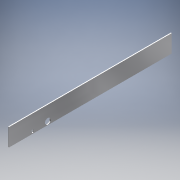
# Autodesk Inventor part: Bumper Plate
Saved by Autodesk Inventor 2019 (Build 230136000, 136)
## iProperties
Created: 2019-10-20
Part Number: Bumper Plate
Material: Aluminum 6061
Document SubType Name: Modeling
Designer: admin
Density: 2.7 g/cm^3
Appearance: Aluminum - Flat
Author: admin
Autodesk Inventor part; units mm, degrees
ref_plane "YZ Plane" through (0, 0, 0) normal (1, 0, 0) x (0, 1, 0)
ref_plane "XZ Plane" through (0, 0, 0) normal (0, 1, 0) x (-1, 0, 0)
ref_plane "XY Plane" through (0, 0, 0) normal (0, 0, 1) x (1, 0, 0)
sketch "Sketch1" plane through (0, 0, 0) normal (1, 0, 0) x (0, 1, 0)
  line L0 (-50, 460) -> (50, 460)
  line L1 (50, 460) -> (50, -460)
  line L2 (50, -460) -> (-50, -460)
  line L3 (-50, -460) -> (-50, 460)
  line L4 (-50, 460) -> (50, -460) construction
  line L5 (50, 460) -> (-50, -460) construction
  point P0 (0, 0)
  dimension "d0" = 920
  dimension "d1" = 100
  constraints: 12 end point, 2 midpoint, 2 parallel, 1 horizontal, 1 perpendicular
  measures "d0" distance of L0.end L1.end
  measures "d1" distance of L0.start L0.end
extrude "Extrusion1" add sketch "Sketch1" along normal blind 5
sketch "Sketch2" plane through (5, 0, 0) normal (1, 0, 0) x (0, 0, -1)
  circle A0 centre (-240.911, -31.452) radius 12.25
  line L0 (-460, -50) -> (460, -50) projected
  line L1 (-460, 50) -> (-460, -50) projected
  point P0 (0, 0)
  dimension "d4" = 24.5
  dimension "d5" = 18.548
  dimension "d8" = 219.089
  constraints: 1 centre point
  measures "d4" diameter of A0
  measures "d5" distance from line of L0 A0.centre
  measures "d8" distance from line of L1 A0.centre
extrude "Extrusion2" cut sketch "Sketch2" against normal through all
sketch "Sketch3" plane through (5, 0, 0) normal (1, 0, 0) x (0, 0, -1)
  arc A0 (-321.8744, -41.3708) -> (-330.8076, -42.4652) centre (-326.341, -41.918) ccw construction
  line L0 (-460, 50) -> (-460, -50) projected
  line L1 (-460, -50) -> (460, -50) projected
  circle A1 centre (-240.911, -31.452) radius 12.25 projected
  arc A2 (-326.9797, -31.4287) -> (-326.341, -41.918) centre (-240.911, -31.452) ccw construction
  arc A3 (-326.8633, -35.9272) -> (-322.4797, -31.4299) centre (-326.9797, -31.4287) ccw construction
  line L2 (-326.9797, -31.4287) -> (-240.911, -31.452) construction
  line L3 (-240.911, -31.452) -> (-326.341, -41.918) construction
  arc A4 (-331.4797, -31.4275) -> (-330.8076, -42.4652) centre (-240.911, -31.452) ccw
  arc A5 (-322.4797, -31.4299) -> (-321.8744, -41.3708) centre (-240.911, -31.452) ccw
  arc A6 (-330.8076, -42.4652) -> (-321.8744, -41.3708) centre (-326.341, -41.918) ccw
  arc A7 (-331.4797, -31.4275) -> (-326.8633, -35.9272) centre (-326.9797, -31.4287) ccw construction
  arc A8 (-322.4797, -31.4299) -> (-331.4797, -31.4275) centre (-326.9797, -31.4287) ccw
  point P0 (0, 0)
  dimension "d9" = 9
  dimension "d10" = 133.659
  dimension "d11" = 8.082
  dimension "d16" = 9
  dimension "d17" = 7
  constraints: 17 point on circle, 8 centre point, 4 coincident, 4 end point, 2 tangent
  measures "d9" diameter of A0
  measures "d10" distance from line of L0 L3.end
  measures "d11" distance from line of L1 L3.end
  measures "d16" diameter of A3
  measures "d17" angle of L3 L2
extrude "Extrusion3" cut sketch "Sketch3" against normal through all contours A8 A5 A6 A4
body "Solid1"
